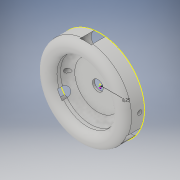
# Autodesk Inventor part: 30_Cube_openSIM_Fouriermask_2
Saved by Autodesk Inventor 2019 (Build 230136000, 136)
## iProperties
Created: 2019-12-02
Part Number: 30_Cube_openSIM_Fouriermask_2
Material: Generic
Document SubType Name: Modeling
Designer: diederichbenedict
Density: 1 g/cm^3
Appearance: Default
Author: diederichbenedict
Autodesk Inventor part; units mm, degrees
ref_plane "YZ Plane" through (0, 0, 0) normal (1, 0, 0) x (0, 1, 0)
ref_plane "XZ Plane" through (0, 0, 0) normal (0, 1, 0) x (-1, 0, 0)
ref_plane "XY Plane" through (0, 0, 0) normal (0, 0, 1) x (1, 0, 0)
sketch "Sketch1" plane through (0, 0, 0) normal (0, 0, 1) x (1, 0, 0)
  circle A0 centre (0, 0) radius 12.5
  circle A1 centre (0, 0) radius 1.5
  dimension "d34" = 25
  dimension "d35" = 3
  constraints: 2 centre point, 1 coincident
  measures "d34" diameter of A0
  measures "d35" diameter of A1
extrude "Extrusion1" add sketch "Sketch1" along normal blind 0.6
sketch "Sketch2" plane through (0, 0, 0.6) normal (0, 0, 1) x (1, 0, 0)
  circle A0 centre (0, 0) radius 12.5 projected
  circle A1 centre (0, 0) radius 8.5
  dimension "d8" = 4
  constraints: 1 centre point
  measures "d8" radial gap between concentric circles of A0 A1
extrude "Extrusion2" add sketch "Sketch2" along normal blind 5
fillet "Fillet1" radius 2 3 edges at (-8.5, 0, 0.6) (-8.5, 0, 5.6) (-12.5, 0, 5.6)
sketch "Sketch3" plane through (0, 0, 0) normal (0, 0, -1) x (-1, 0, 0)
  circle A0 centre (0, 0) radius 12.5 projected
  circle A1 centre (0, -0.75) radius 0.25 projected
  line L0 (-0.2487, -0.7372) -> (-0.25, -0.75)
  line L1 (0, -0.5128) -> (0, -1.0128) construction
  arc A2 (0, -0.5128) -> (-0.2487, -0.7372) centre (0, -0.7628) ccw
  arc A3 (-0.2447, -0.699) -> (0.2447, -0.699) centre (0, -0.75) ccw
  line L2 (0.2487, -0.7372) -> (0.25, -0.75)
  arc A4 (0.2487, -0.7372) -> (0, -0.5128) centre (0, -0.7628) ccw
  point P0 (0, -0.5)
  dimension "d17" = 0.25
  constraints: 10 point on circle, 6 end point, 4 symmetric about line, 3 centre point, 3 coincident, 2 point on line, 1 midpoint, 1 tangent, 7 other
  measures "d17" radius of A2
sketch "Sketch4" plane through (0, 0, 0) normal (0, 0, -1) x (-1, 0, 0)
  circle A0 centre (0, 0) radius 12.5 projected
  circle A1 centre (0, 10.5) radius 2.45
  dimension "d18" = 4.9
  dimension "d19" = 10.5
  constraints: 1 centre point
  measures "d18" diameter of A1
  measures "d19" distance of A0.centre A1.centre
extrude "Extrusion4" cut sketch "Sketch4" against normal blind 4 contours A1 A0 | A0 A1 picked at (-0.073, 11.0129) picked at (0, 12.6429)
pattern_circular "Circular Pattern2" count 3 over 360 about axis through (0, 0, 0) along (0, 0, 1) of "Extrusion4"
sketch "Sketch8" plane through (0, 0, 0) normal (1, 0, 0) x (0, 1, 0)
  line L0 (12.4046, 3.6) -> (-4.8677, 3.6) projected
  line L1 (-4.8677, 0) -> (12.4046, 0) projected
  circle A0 centre (0, 1.3137) radius 0.6099
  line L2 (-4.8677, 0) -> (-4.8677, 3.6) projected
  line L3 (12.4046, 3.6) -> (12.4046, 0) projected
  point P0 (0, 0)
  point P1 (-12.5, 0)
  point P2 (-12.5, 3.6)
  point P3 (12.5, 3.6)
  point P4 (12.5, 0)
  constraints: 1 centre point
extrude "Extrusion6" cut sketch "Sketch8" along normal through all both and the other way through all contours A0
body "Solid1"
